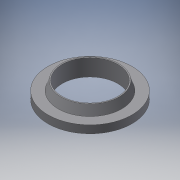
# Autodesk Inventor part: A1-19037-100-XX 28in CL300 Slip on Flange
Saved by Autodesk Inventor 2017.3 (Build 213257000, 257)
## iProperties
Created: 2020-01-21
Part Number: A1-19037-100-XX 28in CL300 Slip on Flange
Material: Generic
Document SubType Name: Modeling
Designer: BEM
Density: 1 g/cm^3
Appearance: Default
Project: A1-19037--CNUL Albian CST laterals
Constructed By: ie_engmgr
Project Name: CST laterals
Author: BEM
Autodesk Inventor part; units mm, degrees
ref_plane "YZ Plane" through (0, 0, 0) normal (1, 0, 0) x (0, 1, 0)
ref_plane "XZ Plane" through (0, 0, 0) normal (0, 1, 0) x (-1, 0, 0)
ref_plane "XY Plane" through (0, 0, 0) normal (0, 0, 1) x (1, 0, 0)
sketch "Sketch1" plane through (0, 0, 0) normal (0, 0, 1) x (1, 0, 0)
  line L0 (0, 0) -> (0, 460.0937) construction
  line L1 (-342.9, 0) -> (-420.0646, 0)
  line L2 (-420.0646, 0) -> (-420.0646, 1.5875)
  line L3 (-420.0646, 1.5875) -> (-342.9, 1.5875)
  line L4 (-342.9, 1.5875) -> (-342.9, 0)
  line L5 (-342.9, 1.5875) -> (-517.525, 1.5875)
  line L6 (-517.525, 1.5875) -> (-517.525, 96.8375)
  line L7 (-517.525, 96.8375) -> (-342.9, 96.8375)
  line L8 (-342.9, 96.8375) -> (-342.9, 1.5875)
  line L9 (-342.9, 96.8375) -> (-342.9, 206.248)
  line L10 (-342.9, 206.248) -> (-355.6, 206.248)
  line L11 (-355.6, 206.248) -> (-391.287, 96.8375)
  dimension "d0" = 342.9
  dimension "d2" = 95.25
  dimension "d3" = 1.5875
  dimension "d4" = 517.525
  dimension "d5" = 206.248
  dimension "d6" = 391.287
  dimension "d7" = 355.6
  constraints: 24 end point, 3 parallel, 3 perpendicular, 2 horizontal, 2 point on line, 2 vertical
  measures "d0" distance between parallel lines of L0 L8
  measures "d2" distance between parallel lines of L5 L7
  measures "d3" distance between parallel lines of L3 L1
  measures "d4" distance between parallel lines of L0 L6
  measures "d5" distance between parallel lines of L1 L10
  measures "d6" distance from line of L11.end L0
  measures "d7" distance from line of L10.end L0
revolve "Revolution1" add sketch "Sketch1" angle 360 about axis through (0, 0, 0) along (0, 1, 0)
body "Solid1"
